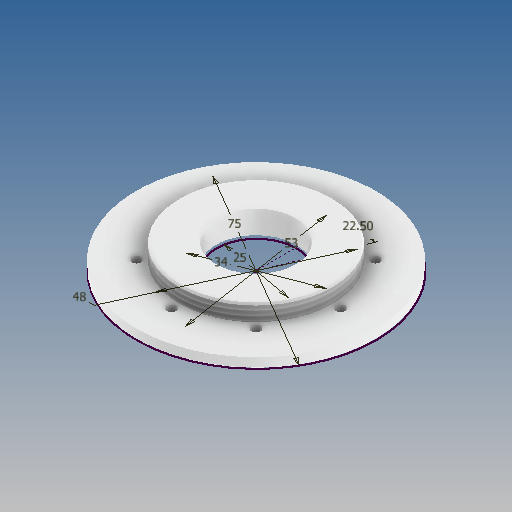
# Autodesk Inventor part: PWTR-0060
Saved by Autodesk Inventor 2021.1 (Build 251245000, 245)
## iProperties
Created: 2020-08-27
Part Number: PWTR-0060
Material: Aluminum 6061
Document SubType Name: Modeling
Designer: alid
Density: 2.7 g/cm^3
Appearance: Aluminum - Flat
Description: Transfer Case Input Cover
Author: alid
Revision Number: A
Autodesk Inventor part; units mm, degrees
ref_plane "YZ Plane" through (0, 0, 0) normal (1, 0, 0) x (0, 1, 0)
ref_plane "XZ Plane" through (0, 0, 0) normal (0, 1, 0) x (-1, 0, 0)
sketch "Sketch1" plane through (0, 0, 0) normal (0, 0, 1) x (1, 0, 0)
  circle A0 centre (0, 0) radius 37.5
  circle A1 centre (0, 0) radius 12.5
  circle A2 centre (0, 0) radius 26.5 construction
  line L0 (0, 0) -> (0, 26.5) construction
  line L1 (0, 0) -> (10.1411, 24.4828) construction
  circle A3 centre (0, 0) radius 24
  circle A4 centre (0, 0) radius 17
  dimension "d0" = 75
  dimension "d1" = 25
  dimension "d2" = 53
  dimension "d3" = 22.5
  dimension "d19" = 48
  dimension "d22" = 34
  constraints: 5 centre point, 5 coincident, 4 end point, 2 point on circle, 1 vertical
  measures "d0" diameter of A0
  measures "d1" diameter of A1
  measures "d2" diameter of A2
  measures "d3" angle of L1 L0
  measures "d19" diameter of A3
  measures "d22" diameter of A4
extrude "Extrusion1" add sketch "Sketch1" along normal blind 3 contours A0 | A3 | A4
extrude "Extrusion2" add sketch "Sketch1" along normal blind 8 contours A3 | A4
chamfer "Chamfer1" distance 0.25 angle 45 1 edges at (-37.5, 0, 0)
ref_plane "Work Plane1" through (-14, -14, 0.8184) normal (0, 0, 1) x (1, 0, 0)
extrude "Extrusion3" cut sketch "Sketch1" along normal up to surface (0.8184 mm away) contours A4
thread "Thread1" size "M48x1.5" class "6g" standard "ISO Metric profile" full length
chamfer "Chamfer2" distance 0.5 angle 45 1 edges at (-24, 0, 8)
hole "Hole2" at (0, 26.5, 0) direction (0, 0, 1) diameter 3 end through all
pattern_circular "Circular Pattern2" count 8 over 360 about axis through (0, 0, -10) along (0, 0, 1) of "Hole2"
body "Solid1"
